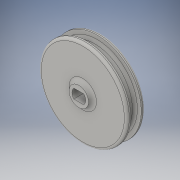
# Autodesk Inventor part: Wheel
Saved by Autodesk Inventor 2016 (Build 200138000, 138)
## iProperties
Created: 2017-09-08
Part Number: Wheel
Material: Generic
Document SubType Name: Modeling
Designer: student
Density: 1 g/cm^3
Appearance: Default
Author: student
Autodesk Inventor part; units mm, degrees
ref_plane "YZ Plane" through (0, 0, 0) normal (1, 0, 0) x (0, 1, 0)
ref_plane "XZ Plane" through (0, 0, 0) normal (0, 1, 0) x (-1, 0, 0)
ref_plane "XY Plane" through (0, 0, 0) normal (0, 0, 1) x (1, 0, 0)
sketch "Sketch8" plane through (0, 0, 0) normal (0, 0, 1) x (1, 0, 0)
  circle A0 centre (0, 0) radius 4.953
  dimension "d46" = 9.906
  constraints: 1 centre point, 1 coincident
  measures "d46" diameter of A0
extrude "Extrusion5" add sketch "Sketch8" along normal blind 2.032
sketch "Sketch9" plane through (0, 0, 0) normal (0, 0, -1) x (-1, 0, 0)
  circle A0 centre (0, 0) radius 22.479
  dimension "d49" = 44.958
  constraints: 1 centre point, 1 coincident
  measures "d49" diameter of A0
extrude "Extrusion6" add sketch "Sketch9" along normal blind 2.032
sketch "Sketch10" plane through (0, 0, -2.032) normal (0, 0, -1) x (-1, 0, 0)
  circle A0 centre (0, 0) radius 19.2405
  dimension "d52" = 38.481
  constraints: 1 centre point, 1 coincident
  measures "d52" diameter of A0
extrude "Extrusion7" add sketch "Sketch10" along normal blind 5.3086
sketch "Sketch11" plane through (0, 0, -7.3406) normal (0, 0, -1) x (-1, 0, 0)
  circle A0 centre (0, 0) radius 22.479
  dimension "d55" = 44.958
  constraints: 1 centre point, 1 coincident
  measures "d55" diameter of A0
extrude "Extrusion8" add sketch "Sketch11" along normal blind 2.032
fillet "Fillet1" radius 1.27 2 edges at (19.2405, 0, -2.032) (19.2405, 0, -7.3406)
sketch "Sketch12" plane through (0, 0, 2.032) normal (0, 0, 1) x (1, 0, 0)
  line L0 (2.5424, 2.413) -> (-2.5424, 2.413)
  line L1 (-2.5424, -2.413) -> (2.5424, -2.413)
  arc A0 (2.5424, -2.413) -> (2.5424, 2.413) centre (0, 0) ccw
  arc A1 (-2.5424, 2.413) -> (-2.5424, -2.413) centre (0, 0) ccw
  constraints: 4 end point, 4 point on circle, 2 centre point, 1 coincident, 1 horizontal, 1 parallel
fillet "Fillet2" radius 2.032 1 edges at (-4.953, 0, 0)
extrude "Extrusion9" cut sketch "Sketch12" against normal blind 5.4864
fillet "Fillet3" radius 1.27 2 edges at (22.479, 0, 0) (22.479, 0, -9.3726)
body "Solid2"
